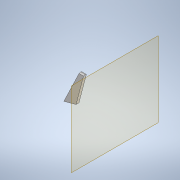
# Autodesk Inventor part: LegConnector
Saved by Autodesk Inventor 2022 (Build 260153000, 153)
## iProperties
Created: 2022-01-06
Part Number: LegConnector
Material: Generic
Document SubType Name: Modeling
Designer: dangl
Density: 1 g/cm^3
Appearance: Default
Author: dangl
Autodesk Inventor part; units mm, degrees
ref_plane "YZ Plane" through (0, 0, 0) normal (1, 0, 0) x (0, 1, 0)
ref_plane "XZ Plane" through (0, 0, 0) normal (0, 1, 0) x (-1, 0, 0)
ref_plane "XY Plane" through (0, 0, 0) normal (0, 0, 1) x (1, 0, 0)
sketch "Sketch1" plane through (0, 0, 0) normal (0, 0, 1) x (1, 0, 0)
  line L0 (-12.7, 177.8) -> (-520.7, 36.275) projected
  line L1 (111.76, 307.9586) -> (-626.11, 307.9586)
  line L2 (-218.6756, 307.9586) -> (-322.6147, 91.4601)
  line L3 (-190.5, 307.9586) -> (-241.3, 114.1137)
  line L4 (-190.5, 307.9586) -> (-218.6756, 307.9586)
  line L5 (-241.3, 114.1137) -> (-322.6147, 91.4601)
  point P0 (0, 0)
  dimension "d0" = 63.5
  dimension "d1" = 25.4
  dimension "d2" = 177.8
  dimension "d3" = 228.6
  constraints: 10 end point, 4 point on line, 1 collinear, 1 horizontal, 2 other
  measures "d0" distance from line of L2 L3.end
  measures "d1" distance from line of L2 L3.start
  measures "d2" horizontal distance of L0.start L3.start
  measures "d3" horizontal distance of L0.start L3.end
extrude "Extrusion1" add sketch "Sketch1" along normal mid plane 19.05
ref_plane "Work Plane1" through (6.35, 234.144, 0) normal (1, 0, 0) x (0, 0, -1)
sketch "Sketch2" plane through (6.35, 234.144, 0) normal (1, 0, 0) x (0, 0, -1)
  line L0 (9.525, 73.8147) -> (-9.525, 73.8147) projected
  line L1 (0, 73.8147) -> (-10.7636, 67.6003)
  line L2 (-10.7636, 67.6003) -> (-10.7636, 77.979)
  line L3 (0, 73.8147) -> (12.8397, 66.4017)
  line L4 (12.8397, 66.4017) -> (12.8397, 77.979)
  line L5 (-10.7636, 77.979) -> (12.8397, 77.979)
  point P0 (0, -234.144)
  dimension "d6" = 120
  dimension "d7" = 60
  dimension "d8" = 60
  constraints: 10 end point, 1 horizontal, 1 midpoint, 1 perpendicular
  measures "d6" angle of L3 L1
  measures "d7" angle of L2 L1
  measures "d8" angle of L4 L3
extrude "Extrusion2" cut sketch "Sketch2" against normal through all
body "Solid1"
